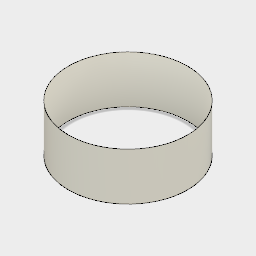
Vertical Thrust Ducts New Version (Autodesk Fusion 360 design; units mm, degrees)
Autodesk Fusion 360 part; units mm, degrees
sketch "Sketch1" plane through (0, 0, 0) normal (0, 0, 1) x (1, 0, 0)
  line L0 (-22.225, 0) -> (-23.8125, 0)
  line L1 (-23.8125, 0) -> (-23.8125, 9.525)
  line L2 (-23.8125, 0) -> (-23.8125, -9.525)
  arc A0 (-23.8125, -9.525) -> (-23.8125, 9.525) centre (-51.5938, 0) ccw
  dimension "d1" = 22.225
  dimension "d2" = 1.5875
  dimension "d3" = 9.525
  dimension "d4" = 9.525
  measures "d1" distance of origin L0.start
  measures "d2" distance of L0.start L0.end
  measures "d3" distance of L0.end L1.end
  measures "d4" distance of L0.end L2.end
sketch "Sketch2" plane through (0, 0, 0) normal (0, 1, 0) x (1, 0, 0)
  circle A0 centre (0, 0) radius 23.8125
  dimension "d5" = 47.625
  measures "d5" diameter of A0
sweep "Sweep1" add profiles "Sketch1" path "Sketch2" along A0 section 1
equation "d2 = ( 1 / 16 ) * 1 in"
equation "d3 = ( 3 / 8 ) * 1 in"
equation "d4 = ( 3 / 8 ) * 1 in"
